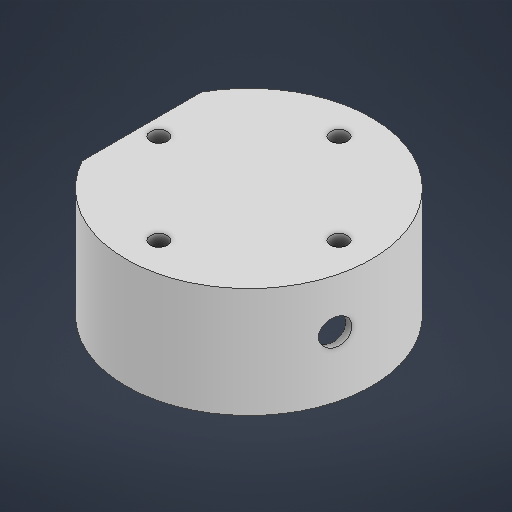
# Autodesk Inventor part: PZT cell
Saved by Autodesk Inventor 2025 (Build 290162000, 162)
## iProperties
Created: 2024-09-13
Part Number: PZT cell
Material: Generic
Document SubType Name: Modeling
Designer: mayhe
Density: 1 g/cm^3
Appearance: Default
Author: mayhe
Autodesk Inventor part; units mm, degrees
ref_plane "YZ Plane" through (0, 0, 0) normal (1, 0, 0) x (0, 1, 0)
ref_plane "XZ Plane" through (0, 0, 0) normal (0, 1, 0) x (-1, 0, 0)
ref_plane "XY Plane" through (0, 0, 0) normal (0, 0, 1) x (1, 0, 0)
sketch "Sketch1" plane through (0, 0, 0) normal (0, 1, 0) x (-1, 0, 0)
  circle A0 centre (0, 0) radius 39.5
  circle A1 centre (0, 0) radius 10
  circle A2 centre (0, 0) radius 29
  circle A3 centre (29, 0) radius 2.75
  circle A4 centre (0, 29) radius 2.75
  circle A5 centre (-29, 0) radius 2.75
  circle A6 centre (0, -29) radius 2.75
  dimension "d2" = 58
  dimension "d0" = 79
  dimension "d1" = 20
  dimension "d3" = 5.5
  dimension "d6" = 360
  constraints: 6 centre point, 3 coincident, 1 horizontal alignment, 11 other
  measures "d0" diameter of A0
  measures "d1" diameter of A1
  measures "d3" diameter of A3
extrude "Extrusion1" add sketch "Sketch1" along normal blind 10 contours A0 | A1 | A3 A2 A6 A5 A4
sketch "Sketch3" plane through (0, 10, 0) normal (0, 1, 0) x (1, 0, 0)
  line L0 (-34.5, 50.157) -> (-34.5, -49.8555)
  circle A0 centre (0, 0) radius 39.5 projected
  point P0 (-34.5, -19.2354)
  point P1 (-34.5, 19.2354)
  dimension "d18" = 5
  constraints: 2 end point, 1 vertical
  measures "d18" distance edge to line of A0 L0
extrude "Extrusion3" cut sketch "Sketch3" along normal through all both and the other way through all contours L0 A0 picked at (-35.5583, 3.956)
sketch "Sketch4" plane through (0, 0, 0) normal (0, -1, 0) x (1, 0, 0)
  circle A0 centre (0, 0) radius 10.16
  dimension "d21" = 20.32
  constraints: 1 centre point, 1 coincident
  measures "d21" diameter of A0
extrude "Extrusion4" cut sketch "Sketch4" against normal blind 3
sketch "Sketch5" plane through (0, 0, 0) normal (0, -1, 0) x (1, 0, 0)
  arc A0 (-34.5, -19.2354) -> (-34.5, 19.2354) centre (0, 0) ccw
  line L0 (-34.5, 19.2354) -> (-34.5, -19.2354) projected
  arc A1 (-32.2183, -19.1893) -> (-32.2183, 19.1893) centre (0, 0) ccw
  circle A2 centre (-29, 0) radius 2.75 projected
  arc A3 (-34.6073, 1.9142) -> (-34.6073, -1.9142) centre (-29, 0) ccw
  arc A4 (-32.7879, 2.2874) -> (-32.7879, -2.2874) centre (-29, 0) ccw
  line L1 (-32.5, -18.1659) -> (-32.5, -3.3212)
  line L2 (-32.5, 3.3212) -> (-32.5, 18.1659)
  line L3 (-34.5, 19.2354) -> (-34.5, 2.5604)
  line L4 (-34.5, -2.5604) -> (-34.5, -19.2354)
  arc A5 (-32.2183, 19.1893) -> (-32.5, 18.1659) centre (-30.5, 18.1659) ccw
  arc A6 (-32.5, -18.1659) -> (-32.2183, -19.1893) centre (-30.5, -18.1659) ccw
  arc A7 (-32.7879, 2.2874) -> (-32.5, 3.3212) centre (-34.5, 3.3212) ccw
  arc A8 (-32.5, -3.3212) -> (-32.7879, -2.2874) centre (-34.5, -3.3212) ccw
  arc A9 (-34.5, -2.5604) -> (-34.6073, -1.9142) centre (-36.5, -2.5604) ccw
  arc A10 (-34.6073, 1.9142) -> (-34.5, 2.5604) centre (-36.5, 2.5604) ccw
  point P0 (-32.5, 18.7083)
  point P1 (-32.5, -18.7083)
  point P2 (-32.5, -2.7075)
  point P3 (-32.5, 2.7075)
  point P4 (-34.5, -2.2035)
  point P5 (-34.5, 2.2035)
  dimension "d24" = 2
  dimension "d25" = 1.5
  dimension "d26" = 2
  dimension "d27" = 2
  constraints: 26 point on circle, 12 tangent, 10 centre point, 8 end point, 7 point on line, 4 equal radius, 2 coincident, 2 collinear
  measures "d24" radial gap between concentric circles of A0 A1
  measures "d25" radial gap between concentric circles of A3 A4
  measures "d26" radius of A5
  measures "d27" radius of A6
extrude "Extrusion5" add sketch "Sketch5" along normal blind 25.4 contours L0 A0 | A9 A3 A10 L0
sketch "Sketch6" plane through (-34.5, 10, -19.2354) normal (-1, 0, 0) x (0, 0, 1)
  circle A0 centre (29.3954, -15.875) radius 4.2498
  point P0 (19.2354, -10)
  constraints: 1 centre point
extrude "Extrusion6" cut sketch "Sketch6" against normal through all
body "Solid1"
